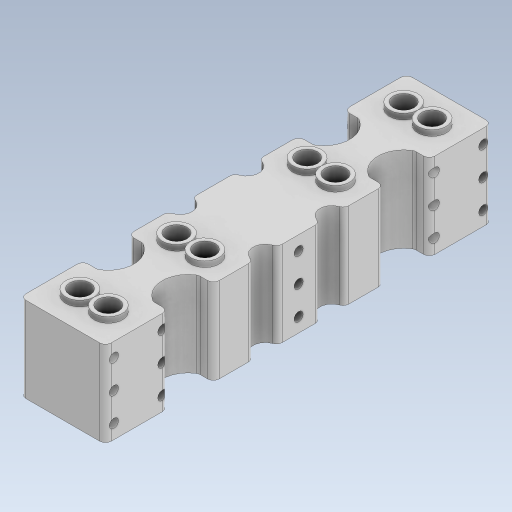
# Autodesk Inventor part: Fix Bracket Gripper
Saved by Autodesk Inventor 2023.5 (Build 275446000, 446)
## iProperties
Created: 2025-10-01
Part Number: Fix Bracket Gripper
Material: Generic
Document SubType Name: Modeling
Designer: Guntur
Density: 1 g/cm^3
Appearance: Default
Author: Guntur
Autodesk Inventor part; units mm, degrees
ref_plane "YZ Plane" through (0, 0, 0) normal (1, 0, 0) x (0, 1, 0)
ref_plane "XZ Plane" through (0, 0, 0) normal (0, 1, 0) x (-1, 0, 0)
ref_plane "XY Plane" through (0, 0, 0) normal (0, 0, 1) x (1, 0, 0)
sketch "Sketch1" plane through (0, 0, 0) normal (0, 1, 0) x (-1, 0, 0)
  line L0 (13, 0) -> (-10.4265, 0) construction
  line L1 (0, 11.6284) -> (0, -16) construction
  line L2 (0, 0) -> (15, 0)
  line L3 (15, 0) -> (15, -5.8286)
  line L4 (15, -7.5) -> (0, -7.5)
  line L5 (0, -7.5) -> (0, 0)
  line L6 (21, 0) -> (-23, 0) construction
  line L7 (0, 19) -> (0, -28) construction
  circle A0 centre (5, -23) radius 3.65
  circle A1 centre (5, -23) radius 5
  circle A2 centre (5, -57) radius 3.65
  circle A3 centre (5, -57) radius 5
  line L8 (0, -16) -> (15, -16)
  line L9 (15, -17.6714) -> (15, -28)
  line L10 (13, -30) -> (10.3483, -30)
  line L11 (0, -30) -> (0, -16)
  line L12 (0, -50) -> (15, -50)
  line L13 (15, -50) -> (15, -64)
  line L14 (15, -64) -> (0, -64)
  line L15 (0, -64) -> (0, -50)
  arc A4 (13.64, -7.7235) -> (13.64, -15.7765) centre (15, -11.75) ccw
  line L16 (15, -50) -> (0, -50)
  line L17 (0, -50) -> (0, -46)
  line L18 (10.3483, -46) -> (13, -46)
  line L19 (15, -48) -> (15, -50)
  line L20 (15, -64) -> (0, -64)
  line L21 (0, -64) -> (0, -68)
  line L22 (0, -68) -> (13, -68)
  line L23 (15, -66) -> (15, -64)
  arc A5 (13.64, -7.7235) -> (15, -5.8286) centre (13, -5.8286) ccw
  arc A6 (15, -17.6714) -> (13.64, -15.7765) centre (13, -17.6714) ccw
  line L24 (-15, 0) -> (-15, -5.8286)
  line L25 (-15, -7.5) -> (0, -7.5)
  circle A7 centre (-5, -23) radius 3.65
  circle A8 centre (-5, -23) radius 5
  circle A9 centre (-5, -57) radius 3.65
  circle A10 centre (-5, -57) radius 5
  line L26 (0, -16) -> (-15, -16)
  line L27 (-15, -17.6714) -> (-15, -28)
  line L28 (-13, -30) -> (-10.3483, -30)
  line L29 (0, -50) -> (-15, -50)
  line L30 (-15, -50) -> (-15, -64)
  line L31 (-15, -64) -> (0, -64)
  arc A11 (-13.64, -15.7765) -> (-13.64, -7.7235) centre (-15, -11.75) ccw
  line L32 (-15, -50) -> (0, -50)
  line L33 (-10.3483, -46) -> (-13, -46)
  line L34 (-15, -48) -> (-15, -50)
  line L35 (-15, -64) -> (0, -64)
  line L36 (0, -68) -> (-13, -68)
  line L37 (-15, -66) -> (-15, -64)
  arc A12 (-15, -5.8286) -> (-13.64, -7.7235) centre (-13, -5.8286) ccw
  arc A13 (-13.64, -15.7765) -> (-15, -17.6714) centre (-13, -17.6714) ccw
  line L38 (0, -11.6284) -> (0, 16) construction
  line L39 (15, 0) -> (15, 5.8286)
  line L40 (15, 7.5) -> (0, 7.5)
  line L41 (0, 7.5) -> (0, 0)
  line L42 (0, -19) -> (0, 28) construction
  circle A14 centre (5, 23) radius 3.65
  circle A15 centre (5, 23) radius 5
  circle A16 centre (5, 57) radius 3.65
  circle A17 centre (5, 57) radius 5
  line L43 (0, 16) -> (15, 16)
  line L44 (15, 17.6714) -> (15, 29)
  line L45 (13, 30) -> (10.3483, 30)
  line L46 (0, 30) -> (0, 16)
  line L47 (0, 50) -> (15, 50)
  line L48 (15, 50) -> (15, 64)
  line L49 (15, 64) -> (0, 64)
  line L50 (0, 64) -> (0, 50)
  arc A18 (13.64, 15.7765) -> (13.64, 7.7235) centre (15, 11.75) ccw
  line L51 (15, 50) -> (0, 50)
  line L52 (0, 50) -> (0, 46)
  line L53 (10.3483, 46) -> (13, 46)
  line L54 (15, 47) -> (15, 50)
  line L55 (15, 64) -> (0, 64)
  line L56 (0, 64) -> (0, 68)
  line L57 (0, 68) -> (13, 68)
  line L58 (15, 66) -> (15, 64)
  arc A19 (15, 5.8286) -> (13.64, 7.7235) centre (13, 5.8286) ccw
  arc A20 (13.64, 15.7765) -> (15, 17.6714) centre (13, 17.6714) ccw
  arc A21 (-15, 17.6714) -> (-13.64, 15.7765) centre (-13, 17.6714) ccw
  circle A22 centre (-5, 23) radius 3.65
  circle A23 centre (-5, 23) radius 5
  line L59 (0, 16) -> (-15, 16)
  arc A24 (-13.64, 7.7235) -> (-13.64, 15.7765) centre (-15, 11.75) ccw
  arc A25 (-13.64, 7.7235) -> (-15, 5.8286) centre (-13, 5.8286) ccw
  line L60 (-15, 7.5) -> (0, 7.5)
  line L61 (-15, 0) -> (-15, 5.8286)
  line L62 (-15, 17.6714) -> (-15, 28)
  line L63 (-13, 30) -> (-10.3483, 30)
  line L64 (-15, 48) -> (-15, 50)
  line L65 (-10.3483, 46) -> (-13, 46)
  line L66 (0, 50) -> (-15, 50)
  line L67 (-15, 50) -> (0, 50)
  line L68 (-15, 50) -> (-15, 64)
  circle A26 centre (-5, 57) radius 3.65
  circle A27 centre (-5, 57) radius 5
  line L69 (-15, 66) -> (-15, 64)
  line L70 (-15, 64) -> (0, 64)
  line L71 (-15, 64) -> (0, 64)
  line L72 (0, 68) -> (-13, 68)
  arc A28 (15, 66) -> (13, 68) centre (13, 66) ccw
  arc A29 (-13, 68) -> (-15, 66) centre (-13, 66) ccw
  arc A30 (13, -68) -> (15, -66) centre (13, -66) ccw
  arc A31 (-15, -66) -> (-13, -68) centre (-13, -66) ccw
  arc A32 (9.2982, 45.7021) -> (9.2982, 30.2979) centre (14.05, 38) ccw
  line L73 (15, 48) -> (15, 47)
  line L74 (15, 28) -> (15, 29)
  arc A33 (13, 46) -> (15, 48) centre (13, 48) ccw
  arc A34 (10.3483, 46) -> (9.2982, 45.7021) centre (10.3483, 44) ccw
  arc A35 (9.2982, 30.2979) -> (10.3483, 30) centre (10.3483, 32) ccw
  arc A36 (15, 28) -> (13, 30) centre (13, 28) ccw
  arc A37 (-9.2982, 30.2979) -> (-9.2982, 45.7021) centre (-14.05, 38) ccw
  line L75 (-15, 47) -> (-15, 46)
  line L76 (-15, 29) -> (-15, 30)
  arc A38 (-9.2982, 45.7021) -> (-10.3483, 46) centre (-10.3483, 44) ccw
  arc A39 (-10.3483, 30) -> (-9.2982, 30.2979) centre (-10.3483, 32) ccw
  arc A40 (-13, 30) -> (-15, 28) centre (-13, 28) ccw
  arc A41 (-15, 48) -> (-13, 46) centre (-13, 48) ccw
  arc A42 (9.2982, -30.2979) -> (9.2982, -45.7021) centre (14.05, -38) ccw
  arc A43 (-9.2982, -45.7021) -> (-9.2982, -30.2979) centre (-14.05, -38) ccw
  line L77 (-15, -29) -> (-15, -30)
  line L78 (-15, -46) -> (-15, -47)
  line L79 (15, -29) -> (15, -30)
  line L80 (15, -46) -> (15, -47)
  arc A44 (13, -30) -> (15, -28) centre (13, -28) ccw
  arc A45 (15, -48) -> (13, -46) centre (13, -48) ccw
  arc A46 (9.2982, -45.7021) -> (10.3483, -46) centre (10.3483, -44) ccw
  arc A47 (10.3483, -30) -> (9.2982, -30.2979) centre (10.3483, -32) ccw
  arc A48 (-10.3483, -46) -> (-9.2982, -45.7021) centre (-10.3483, -44) ccw
  arc A49 (-13, -46) -> (-15, -48) centre (-13, -48) ccw
  arc A50 (-9.2982, -30.2979) -> (-10.3483, -30) centre (-10.3483, -32) ccw
  arc A51 (-15, -28) -> (-13, -30) centre (-13, -28) ccw
  point P0 (15, -68)
  point P1 (-15, -68)
  point P2 (15, 30)
  point P3 (15, 46)
  point P4 (15, 68)
  point P5 (-15, 68)
  point P6 (0, -57)
  point P7 (0, -23)
  point P8 (0, 23)
  point P9 (0, 57)
  point P10 (9.8189, 46)
  point P11 (9.8189, 30)
  point P12 (14.0984, -7.5)
  point P13 (-9.8189, 30)
  point P14 (-9.8189, 46)
  point P15 (9.8189, -30)
  point P16 (9.8189, -46)
  point P17 (-9.8189, -30)
  point P18 (-9.8189, -46)
  dimension "d0" = 15
  dimension "d1" = 7.5
  dimension "d2" = 7.3
  dimension "d3" = 23
  dimension "d4" = 10
  dimension "d6" = 7.3
  dimension "d7" = 10
  dimension "d8" = 34
  dimension "d9" = 4
  dimension "d10" = 4
  dimension "d11" = 2
  dimension "d12" = 2
  dimension "d35" = 2
  dimension "d36" = 2
  dimension "d37" = 2
  constraints: 162 end point, 88 point on circle, 73 symmetric about line, 66 point on line, 52 centre point, 46 tangent, 17 equal radius, 11 parallel, 8 coincident, 7 horizontal, 6 vertical, 5 perpendicular, 4 collinear, 22 other
  measures "d0" distance of L4.start L4.end
  measures "d1" distance of L2.end L4.start
  measures "d2" diameter of A0
  measures "d3" distance from line of L2 A0.centre
  measures "d4" diameter of A1
  measures "d6" diameter of A2
  measures "d7" diameter of A3
  measures "d8" distance of A3.centre A0.centre
  measures "d9" distance of L16.end L17.end
  measures "d10" distance of L21.end L20.end
  measures "d11" radius of A5
  measures "d12" radius of A28
  measures "d35" radius of A33
  measures "d36" radius of A38
  measures "d37" radius of A44
extrude "Extrusion1" add sketch "Sketch1" along normal blind 30 contours L41 L40 A19 L39 L2 | L2 L3 A5 L4 L5 | L5 L25 A12 L24 L61 A25 L60 L41 | L4 A5 A4 A6 L8 L26 A13 A11 A12 L25 | L60 A25 A24 A21 L59 L43 A20 A18 A19 L40 | A6 L9 A44 L10 A47 A42 A46 L18 A45 L19 L12 L29 L34 A49 L33 A48 A43 A50 L28 A51 L27 A13 L26 L8 | L43 L59 A21 L62 A40 L63 A39 A37 A38 L65 A41 L64 L66 L47 L54 A33 L53 A34 A32 A35 L45 A36 L44 A20 | A3 | L13 L14 L15 L12 | A10 | L29 L15 L31 L30 | A17 | L47 L50 L49 L48 | A27 | L68 L70 L50 L66 | L23 A30 L22 L21 L14 | L31 L21 L36 A31 L37 | L49 L56 L57 A28 L58 | L69 A29 L72 L56 L70 | A1 | A8 | A15 | A23
extrude "Extrusion2" add sketch "Sketch1" along normal blind 32 contours A3 | A10 | A17 | A27 | A1 | A8 | A15 | A23
ref_plane "Work Plane1" through (15, 0, 0) normal (1, 0, 0) x (0, 0, -1)
sketch "Sketch2" plane through (15, 0, 0) normal (1, 0, 0) x (0, 0, -1)
  circle A0 centre (0, 25) radius 1.6
  line L0 (-3, 30) -> (3, 30)
  line L1 (-5.8286, 30) -> (5.8286, 30) projected
  line L2 (-5.8286, 0) -> (5.8286, 0) projected
  line L3 (-3, 0) -> (1.6, 0)
  circle A1 centre (0, 5) radius 1.6
  circle A2 centre (-48, 25) radius 1.6
  circle A3 centre (-48, 5) radius 1.6
  circle A4 centre (48, 25) radius 1.6
  circle A5 centre (48, 5) radius 1.6
  circle A6 centre (65, 25) radius 1.6
  circle A7 centre (65, 5) radius 1.6
  circle A8 centre (-65, 25) radius 1.6
  circle A9 centre (-65, 5) radius 1.6
  circle A10 centre (0, 15) radius 1.6
  circle A11 centre (48, 15) radius 1.6
  circle A12 centre (65, 15) radius 1.6
  circle A13 centre (-48, 15) radius 1.6
  circle A14 centre (-65, 15) radius 1.6
  point P0 (0, 0)
  point P1 (-0.7, 0)
  dimension "d17" = 3.2
  dimension "d18" = 3.2
  dimension "d19" = 5
  dimension "d20" = 3.2
  dimension "d21" = 3.2
  dimension "d22" = 3.2
  dimension "d23" = 3.2
  dimension "d26" = 3.2
  dimension "d27" = 3.2
  dimension "d28" = 3.2
  dimension "d29" = 3.2
  dimension "d30" = 3.2
  dimension "d31" = 3.2
  dimension "d32" = 3.2
  dimension "d33" = 3.2
  dimension "d34" = 3.2
  constraints: 15 centre point, 4 end point, 3 point on line, 1 midpoint
  measures "d17" diameter of A0
  measures "d18" diameter of A1
  measures "d19" vertical distance of point (-0.7, 0) A1.centre
  measures "d20" diameter of A2
  measures "d21" diameter of A3
  measures "d22" diameter of A4
  measures "d23" diameter of A5
  measures "d26" diameter of A6
  measures "d27" diameter of A7
  measures "d28" diameter of A8
  measures "d29" diameter of A9
  measures "d30" diameter of A10
  measures "d31" diameter of A11
  measures "d32" diameter of A12
  measures "d33" diameter of A13
  measures "d34" diameter of A14
extrude "Extrusion3" cut sketch "Sketch2" against normal blind 32
body "Solid1"
